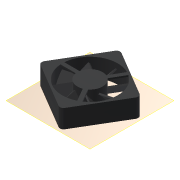
# Autodesk Inventor part: 8025 fan
Saved by Autodesk Inventor 2016 (Build 200138000, 138)
## iProperties
Created: 2018-02-22
Part Number: 8025 fan
Material: ABS Plastic
Document SubType Name: Modeling
Designer: Juny
Density: 1.06 g/cm^3
Appearance: Dark Gray
Author: Juny
Autodesk Inventor part; units mm, degrees
ref_plane "YZ Plane" through (0, 0, 0) normal (1, 0, 0) x (0, 1, 0)
ref_plane "XZ Plane" through (0, 0, 0) normal (0, 1, 0) x (-1, 0, 0)
ref_plane "XY Plane" through (0, 0, 0) normal (0, 0, 1) x (1, 0, 0)
ref_plane "Work Plane1" through (0, 0, 0) normal (0, 0, 1) x (1, 0, 0)
sketch "Sketch1" plane through (0, 0, 0) normal (0, 0, 1) x (1, 0, 0)
  line L0 (13.2065, -51.6751) -> (51.6751, 13.2065) projected
  line L1 (51.6751, 13.2065) -> (-13.2065, 51.6751) projected
  line L2 (-51.6751, -13.2065) -> (13.2065, -51.6751) projected
  line L3 (-13.2065, 51.6751) -> (-51.6751, -13.2065) projected
  line L4 (52.257, 9.706) -> (16.5569, -50.5061)
  line L5 (9.706, -52.257) -> (-50.5061, -16.5569)
  line L6 (-52.257, -9.706) -> (-16.5569, 50.5061)
  line L7 (-9.706, 52.257) -> (50.5061, 16.5569)
  arc A0 (-9.706, 52.257) -> (-16.5569, 50.5061) centre (-12.256, 47.9561) ccw
  arc A1 (52.257, 9.706) -> (50.5061, 16.5569) centre (47.9561, 12.256) ccw
  arc A2 (9.706, -52.257) -> (16.5569, -50.5061) centre (12.256, -47.9561) ccw
  arc A3 (-52.257, -9.706) -> (-50.5061, -16.5569) centre (-47.9561, -12.256) ccw
  point P0 (0, 0)
  dimension "d0" = 80
  dimension "d1" = 5
  constraints: 8 end point, 8 point on circle, 8 tangent, 4 centre point, 3 equal radius, 3 other
  measures "d0" distance between parallel lines of L6 L4
  measures "d1" radius of A0
extrude "Extrusion1" add sketch "Sketch1" along normal blind 25 contours L2 L3 L1 L0 | L4 A2 L5 A3 L6 A0 L7 A1
sketch "Sketch2" plane through (0, 0, 25) normal (0, 0, 1) x (1, 0, 0)
  line L0 (-16.5569, 50.5061) -> (-52.257, -9.706) projected
  arc A0 (-52.257, -9.706) -> (-50.5061, -16.5569) centre (-47.9561, -12.256) ccw projected
  line L1 (-50.5061, -16.5569) -> (9.706, -52.257) projected
  arc A1 (9.706, -52.257) -> (16.5569, -50.5061) centre (12.256, -47.9561) ccw projected
  line L2 (16.5569, -50.5061) -> (52.257, 9.706) projected
  arc A2 (52.257, 9.706) -> (50.5061, 16.5569) centre (47.9561, 12.256) ccw projected
  line L3 (50.5061, 16.5569) -> (-9.706, 52.257) projected
  arc A3 (-9.706, 52.257) -> (-16.5569, 50.5061) centre (-12.256, 47.9561) ccw projected
  circle A4 centre (0, 0) radius 17
  circle A5 centre (0, 0) radius 37.5
  dimension "d4" = 34
  dimension "d5" = 75
  constraints: 2 centre point, 2 coincident
  measures "d4" diameter of A4
  measures "d5" diameter of A5
extrude "Extrusion2" cut sketch "Sketch2" against normal blind 25 contours A5
sketch "Sketch3" plane through (0, 0, 25) normal (0, 0, 1) x (1, 0, 0)
  line L0 (-4.6948, 2.6677) -> (-39.6977, 2.6677)
  line L1 (-39.6977, 2.6677) -> (-39.6977, -2.5088)
  line L2 (-39.6977, -2.5088) -> (-4.6948, -2.5088)
  line L3 (-4.6948, -2.5088) -> (-4.6948, 2.6677)
  point P0 (0, 0)
  constraints: 8 end point, 2 parallel, 1 horizontal, 1 perpendicular
extrude "Extrusion3" add sketch "Sketch3" against normal blind 2
pattern_circular "Circular Pattern1" count 3 over 360 about axis through (0, 0, 25) along (0, 0, -1) of "Extrusion3"
sketch "Sketch4" plane through (52.257, 9.706, 25) normal (0.8601734, -0.5100017, 0) x (0, 0, -1)
  line L0 (22.2917, -28.6045) -> (5.6369, -42.5796)
  line L1 (5.6369, -42.5796) -> (6.8927, -44.0763)
  line L2 (6.8927, -44.0763) -> (23.5476, -30.1012)
  line L3 (23.5476, -30.1012) -> (22.2917, -28.6045)
  line L4 (25, -70) -> (25, 0) projected
  point P0 (25, -35)
  dimension "d13" = 50
  constraints: 8 end point, 2 parallel, 1 perpendicular
  measures "d13" angle of L4 L0
extrude "Extrusion4" add sketch "Sketch4" against normal up to surface separate body round surface about axis through (0, 0, 25) along (0, 0, -1) radius 17 far side no
pattern_circular "Circular Pattern2" count 8 over 360 about axis through (0, 0, 25) along (0, 0, -1) of "Extrusion4" bodies 2
sketch "Sketch5" plane through (0, 0, 25) normal (0, 0, 1) x (1, 0, 0)
  circle A0 centre (0, 0) radius 36.4881
  circle A1 centre (0, 0) radius 45.6015
  constraints: 2 centre point, 2 coincident
extrude "Extrusion5" cut sketch "Sketch5" against normal blind 40 bodies 2
body "Solid1"
body "Solid2"
